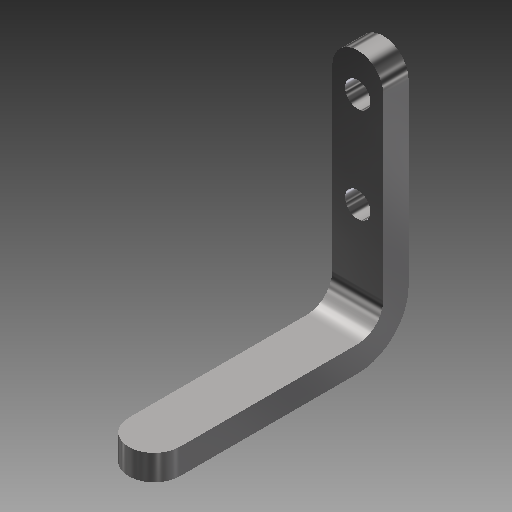
# Autodesk Inventor part: Pręt_łączący
Saved by Autodesk Inventor 2017 (Build 210142000, 142)
## iProperties
Created: 2015-12-05
Part Number: Pręt_łączący
Material: Stal nierdzewna
Document SubType Name: Sheet Metal
Designer: graaapsik
Density: 8.08 g/cm^3
Sheet Metal Rule: Default_mm
Appearance: Częściowo polerowany
Sheet Metal Width: 0,000 mm
Sheet Metal Length: 0,000 mm
Sheet Metal Area: 0,000 mm^2
Mass: 34.626 g
Surface Area: 28.4613 cm^2
Volume: 4.2854 cm^3
Author: graaapsik
Autodesk Inventor part; units mm, degrees
ref_plane "YZ Plane" through (0, 0, 0) normal (1, 0, 0) x (0, 1, 0)
ref_plane "XZ Plane" through (0, 0, 0) normal (0, 1, 0) x (-1, 0, 0)
ref_plane "XY Plane" through (0, 0, 0) normal (0, 0, 1) x (1, 0, 0)
sketch "Szkic1" plane through (0, 0, 0) normal (0, 0, 1) x (1, 0, 0)
  line L0 (0, 0) -> (10, 0)
  line L1 (10, 0) -> (10, 50)
  line L2 (10, 50) -> (0, 50)
  line L3 (0, 50) -> (0, 0)
  dimension "d0" = 50
  dimension "d1" = 10
  measures "d0" distance of L0.end L1.end
  measures "d1" distance of L0.start L0.end
extrude "Płyta1" add sketch "Szkic1" along normal blind 5
sketch "Szkic3" plane through (10, 5, 0) normal (0, -1, 0) x (1, 0, 0)
  line L0 (-10, 0) -> (0, 0)
  line L1 (0, 0) -> (0, 50)
  line L2 (0, 50) -> (-10, 50)
  line L3 (-10, 50) -> (-10, 0)
  constraints: 6 end point, 1 horizontal, 1 perpendicular, 1 vertical
edge flange "Kołnierz1" height 50 angle 90 thickness 5 bend radius 5 thickness toward (0, -1, 0) relief tear relief width 5 relief depth 2.5 edges at (5, 0, 5) wall of the first edge with corners at (0, 5, 0) (10, 5, 0) (10, 5, 50) (0, 5, 50)
bend "Gięcie1"
corner "Narożnik1"
sketch "Szkic2" plane through (0, 0, 5) normal (0, 0, 1) x (1, 0, 0)
  line L0 (0, 0) -> (0, 50) construction
  line L1 (10, 50) -> (10, 0) construction
  arc A0 (10, 45) -> (0, 45) centre (5, 45) ccw
  line L2 (5, 23.75) -> (5.65, 23.75) construction
  point P0 (5, 42.5)
  point P1 (5, 5)
  point P2 (0, 5)
  point P3 (10, 5)
  dimension "d5" = 5
  dimension "d6" = 5
  dimension "d7" = 2.5
  constraints: 6 end point, 2 point on circle, 2 vertical alignment, 1 centre point, 1 perpendicular, 1 symmetric about line
  measures "d5" horizontal distance of point (5, 5) L0.start
  measures "d6" horizontal distance of L0.start point (5, 5)
  measures "d7" distance of A0.centre point (5, 42.5)
hole "Otwór4" at (5, 42.5, 5) at (5, 23.75, 5) direction (0, 0, -1) diameter 5 end through all
fillet "Zaokrąglenie2" radius 5 4 edges at (0, 2.5, 50) (10, 2.5, 50) (10, 50, 2.5) (0, 50, 2.5)
equation "\"d45\" = Grubość"
equation "\"d23\" = SzerokośćGięciaPodcięcia"
equation "\"d24\" = GłębokośćGięciaPodcięcia"
equation "\"d25\" = MinimalnaPozostałość"
equation "\"d26\" = PromieńGięcia"
equation "\"d29\" = PromieńGięcia"
equation "\"d30\" = RozmiarPodcięciaNarożnika"
equation "\"d31\" = Wielk_odstępu"
equation "\"d32\" = Rozmiar_promienia_Jacobiego"
equation "\"PromieńGięcia\" = Grubość"
equation "\"SzerokośćGięciaPodcięcia\" = Grubość"
equation "\"GłębokośćGięciaPodcięcia\" = 0.5 * Grubość"
equation "\"PromieńPrzejścia\" = PromieńGięcia"
equation "\"Rozmiar_promienia_Jacobiego\" = PromieńGięcia"
equation "\"Wielk_odstępu\" = Grubość"
equation "\"d2\" = PromieńGięcia"
equation "\"Grubość\" = 5"
equation "\"MinimalnaPozostałość\" = 10"
equation "\"RozmiarPodcięciaNarożnika\" = 20"
